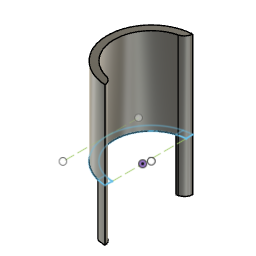
Dome (Autodesk Fusion 360 design; units mm, degrees)
Autodesk Fusion 360 part; units mm, degrees
sketch "Sketch3" plane through (0, 0, 0) normal (0, 0, 1) x (1, 0, 0)
  arc A0 (0, 5) -> (0, -3.5) centre (0.2386, 0.75) ccw
  arc A1 (-0.0448, 5.7987) -> (-0.0448, -4.2987) centre (0.2386, 0.75) ccw
  line L0 (-0.0448, 5.7987) -> (0, 5)
  line L1 (0, -3.5) -> (-0.0448, -4.2987)
  line L2 (0, 5) -> (0, -3.5) construction
  line L3 (-4.8181, 4.3421) -> (-4.8181, -4.3593) construction
  line L4 (-0.9977, -4.1533) -> (-0.9977, -3.3232)
  line L5 (-0.9977, 4.8232) -> (-0.9977, 5.6533)
  dimension "d2" = 0.8
  dimension "d17" = 8.5
  constraint vertical A0.start A0.end
  constraint tangent A1 L3
  constraint vertical L3
  constraint coincident A1 L4.start
  constraint coincident A0 L4.end
  constraint vertical L4
  constraint coincident A0 L5.start
  constraint coincident A1 L5.end
  constraint parallel L4 L5
  measures "d17" distance of A0.start A0.end
extrude "Extrude1" add sketch "Sketch3" along normal blind 10
fillet "Fillet1" radius 1 1 edges at (0, -3.5, 5)
fillet "Fillet2" radius 1 1 edges at (0, 5, 5)
extrude "Extrude2" add sketch "Sketch3" against normal blind 6 contours A0 A1 L1 L4
fillet "Fillet3" radius 1 1 edges at (0, -3.5, -3)
extrude "Extrude3" add sketch "Sketch3" against normal blind 6 contours A0 A1 L0 L5
fillet "Fillet4" radius 1 1 edges at (0, 5, -3)
sketch "Sketch2" plane through (0, 0, 0) normal (0, 0, 1) x (1, 0, 0)
  arc A0 (29, 28) -> (29, 0) centre (33.35, 14) ccw
